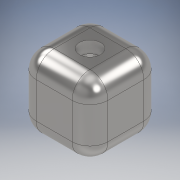
# Autodesk Inventor part: Part5
Saved by Autodesk Inventor 2020 (Build 240168000, 168)
## iProperties
Created: 2021-11-29
Part Number: Part5
Material: Steel, Alloy
Document SubType Name: Modeling
Designer: Emrah BAYRAM
Density: 7.73 g/cm^3
Appearance: Semi-Polished
Mass: 161.272 g
Surface Area: 49.6283 cm^2
Volume: 20.8631 cm^3
Author: Emrah BAYRAM
Autodesk Inventor part; units mm, degrees
ref_plane "YZ Plane" through (0, 0, 0) normal (1, 0, 0) x (0, 1, 0)
ref_plane "XZ Plane" through (0, 0, 0) normal (0, 1, 0) x (-1, 0, 0)
ref_plane "XY Plane" through (0, 0, 0) normal (0, 0, 1) x (1, 0, 0)
sketch "Sketch1" plane through (0, 0, 0) normal (0, 1, 0) x (-1, 0, 0)
  line L0 (0, 0) -> (-30, 0)
  line L1 (-30, 0) -> (-30, -30)
  line L2 (-30, -30) -> (0, -30)
  line L3 (0, -30) -> (0, 0)
  dimension "d0" = 30
  dimension "d1" = 30
  constraints: 8 end point, 2 parallel, 1 horizontal, 1 perpendicular
  measures "d0" distance of L2.end L1.end
  measures "d1" distance of L1.end L0.end
extrude "Extrusion1" add sketch "Sketch1" along normal blind 30
sketch "Sketch2" plane through (0, 30, 0) normal (0, 1, 0) x (1, 0, 0)
  line L0 (30, 30) -> (0, 30) projected
  line L1 (0, 30) -> (0, 0) projected
  line L2 (0, 0) -> (30, 0) projected
  line L3 (30, 0) -> (30, 30) projected
  circle A0 centre (15, 15) radius 5
  dimension "d4" = 10
  dimension "d13" = 15
  dimension "d14" = 15
  constraints: 1 centre point
  measures "d4" diameter of A0
  measures "d13" distance from line of L2 A0.centre
  measures "d14" distance from line of L1 A0.centre
hole "Hole1" at (15, 30, -15) direction (0, -1, 0) diameter 8.8 depth 5 tip angle 118
fillet "Fillet2" radius 7.5 12 edges at (0, 30, -15) (15, 30, -30) (30, 30, -15) (15, 30, 0) (30, 15, -30) (30, 15, 0) (30, 0, -15) (15, 0, -30) (0, 15, -30) (15, 0, 0) (0, 15, 0) (0, 0, -15)
body "Solid1"
